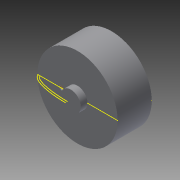
# Autodesk Inventor part: data_logger
Saved by Autodesk Inventor 2015 (Build 190159000, 159)
## iProperties
Created: 2019-09-28
Part Number: data_logger
Material: Generic
Document SubType Name: Modeling
Designer: gabri
Density: 1 g/cm^3
Appearance: Default
Author: gabri
Autodesk Inventor part; units mm, degrees
ref_plane "YZ Plane" through (0, 0, 0) normal (1, 0, 0) x (0, 1, 0)
ref_plane "XZ Plane" through (0, 0, 0) normal (0, 1, 0) x (-1, 0, 0)
ref_plane "XY Plane" through (0, 0, 0) normal (0, 0, 1) x (1, 0, 0)
sketch "Sketch2" plane through (0, 0, 0) normal (0, 0, 1) x (1, 0, 0)
  line L0 (0, -5) -> (-6, -5)
  line L1 (-6, -5) -> (-6, 0)
  line L2 (-30, -1.5) -> (-30, 0)
  line L3 (-7.5, -1.5) -> (-7.5, -6.5)
  line L4 (-7.5, -6.5) -> (0, -6.5)
  line L5 (-27, 0) -> (-27, 24)
  line L6 (-27, 24) -> (-30, 24)
  line L7 (-30, 24) -> (-30, 0)
  line L8 (-7.5, -1.5) -> (-30, -1.5)
  line L9 (-27, 0) -> (-6, 0)
  line L10 (0, -5) -> (0, -6.5)
  point P0 (0, 0)
  dimension "d16" = 1.5
  dimension "d18" = 1.5
  dimension "d21" = 3
  dimension "d22" = 24
  dimension "d51" = 5
  dimension "d52" = 1.5
  dimension "d53" = 1.5
  constraints: 22 end point, 2 parallel, 1 horizontal, 1 perpendicular, 1 vertical
  measures "d16" distance of L2.start L2.end
  measures "d18" distance between parallel lines of L3 L1
  measures "d21" distance of L5.end L6.end
  measures "d22" distance of L6.end L2.end
  measures "d51" distance between parallel lines of L9 L0
  measures "d52" distance between parallel lines of L8 L9
  measures "d53" distance of L0.start L4.end
revolve "Revolution1" add sketch "Sketch2" angle 360 about axis through (0, -5, 0) along (0, -1, 0)
sketch "Sketch4" plane through (0, 0, 0) normal (0, 1, 0) x (1, 0, 0)
  circle A0 centre (0, 0) radius 6 projected
  line L0 (-27, 1.5) -> (27, 1.5)
  line L1 (27, 1.5) -> (27, -1.5)
  line L2 (27, -1.5) -> (-27, -1.5)
  line L3 (-27, -1.5) -> (-27, 1.5)
  point P0 (0, 0)
  dimension "d28" = 1.5
  dimension "d29" = 3
  dimension "d30" = 27
  dimension "d31" = 27
  constraints: 8 end point, 2 parallel, 1 horizontal, 1 perpendicular
  measures "d28" distance from line of point (0, 0) L0
  measures "d29" distance of L0.end L1.end
  measures "d30" distance from line of point (0, 0) L3
  measures "d31" distance from line of point (0, 0) L1
extrude "Extrusion1" cut sketch "Sketch4" along normal blind 24 and the other way blind 0.5 contours A0 L2 L0 | A0 L0 L1 L2 | A0 L2 L3 L0
sketch "Sketch5" plane through (27, -0.5, -1.5) normal (-1, 0, 0) x (0, 0, 1)
  line L0 (3, 24.5) -> (0, 24.5)
  line L1 (0, 24.5) -> (0, 0.5)
  line L2 (0, 0.5) -> (3, 0.5)
  line L3 (3, 0.5) -> (3, 24.5)
  line L4 (31.5, 24.5) -> (-28.5, 24.5) projected
  point P0 (1.5, 0.5)
  point P1 (1.5, 0.5)
  dimension "d36" = 3
  dimension "d37" = 0
  constraints: 8 end point, 2 parallel, 1 coincident, 1 horizontal, 1 midpoint, 1 perpendicular
  measures "d36" distance of L1.end L2.end
  measures "d37" distance between parallel lines of L4 L0
extrude "Extrusion2" cut sketch "Sketch5" against normal blind 1
sketch "Sketch6" plane through (-27, -0.5, 1.5) normal (1, 0, 0) x (0, 0, -1)
  line L0 (0, 0.5) -> (3, 0.5)
  line L1 (3, 0.5) -> (3, 24.5)
  line L2 (3, 24.5) -> (0, 24.5)
  line L3 (0, 24.5) -> (0, 0.5)
  line L4 (31.5, 24.5) -> (-28.5, 24.5) projected
  point P0 (1.5, 0.5)
  point P1 (1.5, 0.5)
  point P2 (1.5, 24.5)
  dimension "d40" = 3
  constraints: 8 end point, 3 midpoint, 2 parallel, 1 coincident, 1 horizontal, 1 perpendicular
  measures "d40" distance between parallel lines of L1 L3
extrude "Extrusion3" cut sketch "Sketch6" against normal blind 1
sketch "Sketch7" plane through (0, -0.5, 0) normal (0, 1, 0) x (1, 0, 0)
  point P0 (0, 0)
  point P1 (-12, 0)
  dimension "d43" = 12
  measures "d43" distance of point (0, 0) point (-12, 0)
hole "Hole1" at (-12, -0.5, 0) direction (0, -1, 0) diameter 3 end through all
ref_plane "Work Plane1" through (-26.958301, 0, 0) normal (0, 0, 1) x (1, 0, 0)
sketch "Sketch10" plane through (-26.958301, 0, 0) normal (0, 0, 1) x (1, 0, 0)
  line L0 (56.958301, -1.5) -> (-3.041699, -1.5)
  line L1 (56.958301, -1.5) -> (-3.041699, -1.5)
  line L2 (26.958301, -1.5) -> (26.958301, -8)
  line L3 (-1.541699, -1.5) -> (0.458301, -1.5)
  line L4 (4.493832, -1.5) -> (4.493832, -5.5)
  ellipse E0 centre (26.958301, -1.5) end of major axis (-1.541699, -1.5) minor radius 6.5
  line L5 (0.458301, -1.5) -> (4.493832, -1.5)
  point P0 (26.958301, 0)
  dimension "d67" = 28.5
  dimension "d56" = 6.5
  dimension "d65" = 4
  constraints: 8 end point, 3 point on line, 2 vertical, 1 coincident, 1 collinear, 1 horizontal, 1 midpoint, 5 other
  measures "d56" distance of L2.start L2.end
  measures "d65" distance of L4.start L4.end
revolve "Revolution3" add sketch "Sketch10" angle 5 about axis through (0, -1.5, 0) along (0, -1, 0) and the other way 5 contours L4 E0 L0
sketch "Sketch12" plane through (-22.378985, -5.5, 1.957907) normal (0.0871557, 0, 0.9961947) x (0.9961947, 0, -0.0871557)
  line L0 (0, 4) -> (0.341286, 4)
  line L1 (0.341286, 4) -> (0.341286, 0)
  line L2 (0.341286, 0) -> (0, 0)
  line L3 (0, 0) -> (0, 4)
  point P0 (22.464469, 5.5)
  constraints: 8 end point, 2 parallel, 1 horizontal, 1 perpendicular
extrude "Extrusion5" cut sketch "Sketch12" against normal through all
sketch "Sketch13" plane through (-22.378985, -5.5, 1.957907) normal (0.9961947, 0, -0.0871557) x (-0.0871557, 0, -0.9961947)
  line L0 (0, 4) -> (0, 0)
  line L1 (4.948973, 4) -> (0, 4)
  ellipse E0 centre (0, 4) end of major axis (0, 10.5) minor radius 4.948973 (3.961092, 0.103353) -> (4.948973, 4) ccw
  line L2 (0, 4) -> (0, 0)
  line L3 (0, 0) -> (0, 4)
  line L4 (0.858913, 5) -> (3.847497, 5)
  line L5 (1.986817, 5) -> (1.986817, 0.025749)
  point P0 (0, 5.5)
  point P1 (1.986817, 2)
  dimension "d72" = 2
  dimension "d74" = 0
  constraints: 2 end point, 1 perpendicular, 1 point on line, 3 other
  measures "d72" distance from line of L1 point (1.987, 2)
  measures "d74" distance from line of L5 point (1.987, 2)
hole "Hole2" at (-22.552147, -3.5, -0.02135) direction (-0.9961947, 0, 0.0871557) diameter 2 end through all
pattern_circular "Circular Pattern1" count 4 over 360 about axis through (0, -4, 0) along (0, 1, 0) of "Revolution3", "Extrusion5", "Hole2"
equation "\"d18\" = d16"
equation "\"d29\" = 2 * d28"
body "Solid1"
